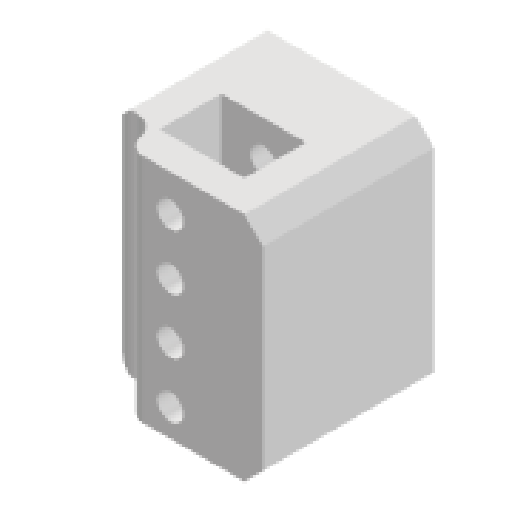
# Autodesk Inventor part: OT2-Gripper_block
Saved by Autodesk Inventor 2024.1 (Build 281209000, 209)
## iProperties
Created: 2024-09-05
Part Number: OT2-Gripper_block
Material: Generisch
Document SubType Name: Modeling
Designer: diederichbenedict
Density: 1 g/cm^3
Appearance: Vorgabe
Author: diederichbenedict
Autodesk Inventor part; units mm, degrees
ref_plane "YZ Plane" through (0, 0, 0) normal (1, 0, 0) x (0, 1, 0)
ref_plane "XZ Plane" through (0, 0, 0) normal (0, 1, 0) x (-1, 0, 0)
ref_plane "XY Plane" through (0, 0, 0) normal (0, 0, 1) x (1, 0, 0)
sketch "Skizze1" plane through (0, 0, 0) normal (0, 0, 1) x (1, 0, 0)
  line L0 (-4.5, 3.25) -> (-4.5, 2.25) projected
  arc A0 (-3.564, 1.602) -> (-4.5, 2.25) centre (-4.5, 1.25) ccw projected
  line L1 (-3.564, 1.602) -> (-3.2351, 1.602) projected
  line L2 (-3.2351, 1.602) -> (-3.2351, 0.898) projected
  line L3 (-3.2351, 0.898) -> (-3.564, 0.898) projected
  arc A1 (-4.5, 0.25) -> (-3.564, 0.898) centre (-4.5, 1.25) ccw projected
  line L4 (-4.5, 0.25) -> (-4.5, -3.25) projected
  line L5 (-4.5, -3.25) -> (4.5, -3.25) projected
  line L6 (4.5, -3.25) -> (4.5, 0.25) projected
  arc A2 (3.564, 0.898) -> (4.5, 0.25) centre (4.5, 1.25) ccw projected
  line L7 (3.564, 0.898) -> (3.2351, 0.898) projected
  line L8 (3.2351, 0.898) -> (3.2351, 1.602) projected
  line L9 (3.2351, 1.602) -> (3.564, 1.602) projected
  arc A3 (4.5, 2.25) -> (3.564, 1.602) centre (4.5, 1.25) ccw projected
  line L10 (4.5, 2.25) -> (4.5, 3.25) projected
  line L11 (4.5, 3.25) -> (-4.5, 3.25) projected
  line L12 (4.575, -3.325) -> (-4.575, -3.325)
  line L13 (-4.575, -3.325) -> (-4.575, 0.328)
  arc A4 (-4.575, 0.328) -> (-3.6174, 0.973) centre (-4.5, 1.25) ccw
  line L14 (-3.6174, 0.973) -> (-3.3101, 0.973)
  line L15 (-3.3101, 0.973) -> (-3.3101, 1.527)
  line L16 (-3.3101, 1.527) -> (-3.6174, 1.527)
  arc A5 (-3.6174, 1.527) -> (-4.575, 2.172) centre (-4.5, 1.25) ccw
  line L17 (-4.575, 2.172) -> (-4.575, 3.325)
  line L18 (-4.575, 3.325) -> (4.575, 3.325)
  line L19 (4.575, 3.325) -> (4.575, 2.172)
  arc A6 (4.575, 2.172) -> (3.6174, 1.527) centre (4.5, 1.25) ccw
  line L20 (3.6174, 1.527) -> (3.3101, 1.527)
  line L21 (3.3101, 1.527) -> (3.3101, 0.973)
  line L22 (3.3101, 0.973) -> (3.6174, 0.973)
  arc A7 (3.6174, 0.973) -> (4.575, 0.328) centre (4.5, 1.25) ccw
  line L23 (4.575, 0.328) -> (4.575, -3.325)
  circle A8 centre (-15.1, -13.35) radius 3.5 projected
  line L24 (-20.2, -17.25) -> (-22.2, -15.25) projected
  line L25 (-20.2, -17.25) -> (9.8, -17.25) projected
  line L26 (9.8, -17.25) -> (9.8, 6.75) projected
  line L27 (-11.8, 6.75) -> (9.8, 6.75) projected
  line L28 (-11.8, 11.75) -> (-11.8, 6.75) projected
  line L29 (-20.2, 11.75) -> (-11.8, 11.75) projected
  line L30 (-22.2, 9.75) -> (-20.2, 11.75) projected
  line L31 (-22.2, -15.25) -> (-22.2, 9.75) projected
  line L32 (-11.8, 6.75) -> (-9.8, 6.75) projected
  line L33 (-9.8, 6.75) -> (-9.8, 11.75) projected
  line L34 (-9.8, 11.75) -> (-11.8, 11.75) projected
  line L35 (-11.8, 11.75) -> (-11.8, 6.75) projected
  line L36 (9.8, 11.75) -> (-20.2, 11.75) projected
  circle A9 centre (-15.1, -13.35) radius 1.1 projected
  line L37 (-22.2, -15.25) -> (-20.2, -17.25) projected
  line L38 (-22.2, -15.25) -> (-22.2, 9.75) projected
  line L39 (-20.2, 11.75) -> (-22.2, 9.75) projected
  line L40 (9.8, 11.75) -> (-20.2, 11.75) projected
  line L41 (9.8, -17.25) -> (9.8, 11.75) projected
  line L42 (9.8, -17.25) -> (-20.2, -17.25) projected
  line L43 (-10, 6.75) -> (10, 6.75)
  line L44 (10, 6.75) -> (10, -6.75)
  line L45 (10, -6.75) -> (-10, -6.75)
  line L46 (-10, -6.75) -> (-10, 6.75)
  line L47 (-10, 6.75) -> (10, -6.75) construction
  line L48 (10, 6.75) -> (-10, -6.75) construction
  line L49 (10, 6.75) -> (-10, 6.75)
  line L50 (-10, 6.75) -> (-10, 11.75)
  line L51 (-10, 11.75) -> (10, 11.75)
  line L52 (10, 11.75) -> (10, 6.75)
  line L53 (-4.575, 0.328) -> (-4.575, 2.172)
  line L54 (4.575, 0.328) -> (4.575, 2.172)
  line L55 (9.8, 11.75) -> (-20.2, 11.75) projected
  point P0 (0, 0)
  point P1 (4.5, -1.5)
  point P2 (4.575, -1.4985)
  dimension "d0" = 0.075
  dimension "d1" = 20
  dimension "d2" = 13.5
  constraints: 48 end point, 8 point on circle, 4 centre point, 4 midpoint, 4 parallel, 2 horizontal, 2 perpendicular, 2 vertical, 1 point on line, 15 other
  measures "d0" distance of point (4.5, -1.5) point (4.575, -1.498)
  measures "d1" distance of L44.end L45.end
  measures "d2" distance of L43.end L44.end
extrude "Extrusion1" add sketch "Skizze1" along normal blind 25 contours L45 L46 L27 L26 | L26 L43 L44 L45 | L27 L33 L36 L41 | L41 L51 L52 L43 | L27 L50 L34 L33
sketch "Skizze2" plane through (-10, 11.75, 0) normal (0, 1, 0) x (1, 0, 0)
  line L0 (20, 0) -> (0, 0) projected
  line L1 (0, 0) -> (0, -25) projected
  line L2 (20, -25) -> (0, -25) projected
  line L3 (20, 0) -> (20, -25) projected
  line L4 (10, -12.6) -> (10, 75.6)
  point P0 (10, 0)
  point P1 (10, -3)
  dimension "d5" = 3
  constraints: 2 end point, 1 point on line, 1 vertical, 2 other
  measures "d5" distance from line of point (10, -3) L0
hole "Bohrung1" at (0, 11.75, 3) direction (0, -1, 0) diameter 2.8 end through all
pattern_linear "Rechteckige Anordnung1" count 4 spacing 6 along (0, 0, 1) of "Bohrung1"
chamfer "Fasen1" distance 2 angle 45 4 edges at (-10, 2.5, 0) (-10, 2.5, 25) (10, 2.5, 0) (10, 2.5, 25)
sketch "Skizze3" plane through (0, 0, 25) normal (0, 0, 1) x (1, 0, 0)
  line L0 (-5, -18.15) -> (-5, -21.15) projected
  line L1 (-22.9, -3.25) -> (-19.9, -3.25) projected
  circle A0 centre (-15.1, -13.35) radius 1.4224 projected
  line L2 (-5, -5.55) -> (-5, -8.55) projected
  arc A1 (-5, -5.55) -> (-7.3, -3.25) centre (-7.3, -5.55) ccw projected
  line L3 (-10.3, -3.25) -> (-7.3, -3.25) projected
  line L4 (-25.2, -23.45) -> (-5, -23.45)
  line L5 (-5, -23.45) -> (-5, -3.25)
  line L6 (-5, -3.25) -> (-25.2, -3.25)
  line L7 (-25.2, -3.25) -> (-25.2, -23.45)
  line L8 (-25.2, -23.45) -> (-5, -3.25) construction
  line L9 (-5, -23.45) -> (-25.2, -3.25) construction
  line L10 (-10.3, -3.1) -> (-7.3, -3.1)
  arc A2 (-4.85, -5.55) -> (-7.3, -3.1) centre (-7.3, -5.55) ccw
  line L11 (-4.85, -5.55) -> (-4.85, -8.55)
  line L12 (-4.85, -3.1) -> (-4.85, -23.6)
  line L13 (-4.85, -23.6) -> (-25.35, -23.6)
  line L14 (-25.35, -23.6) -> (-25.35, -3.1)
  line L15 (-25.35, -3.1) -> (-4.85, -3.1)
  point P0 (0, 0)
  dimension "d19" = 0.15
  constraints: 24 end point, 4 parallel, 2 midpoint, 2 perpendicular, 2 point on circle, 1 centre point, 1 horizontal, 1 point on line, 5 other
  measures "d19" radial gap between concentric circles of A1 A2
extrude "Extrusion2" cut sketch "Skizze3" against normal blind 25 contours L5 L2 A2 L11 L12 L13 L14 L15 L10 L6 L3 L1 L7 L4 L0 | L0 L5 L4 L7 L6 L1 L3 A1 L2 | A1 L6 A2 L5
fillet "Rundung1" radius 2 2 edges at (-4.85, -6.75, 12.5) (-10, -3.1, 12.5)
